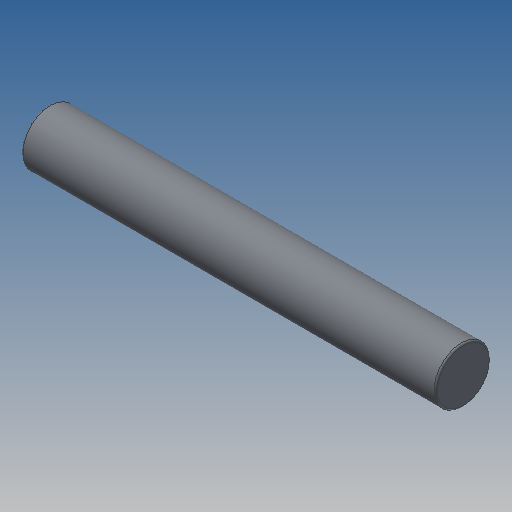
# Autodesk Inventor part: 87994-LtBluishGray
Saved by Autodesk Inventor 2022.2 (Build 262287010, 287A)
## iProperties
Created: 2014-06-03
Part Number: 87994-LtBluishGray
Material: ABS Plastic
Document SubType Name: Modeling
Designer: D. Kohfeld
Appearance: LtBluishGray
Mass: 0.204556 g
Surface Area: 2.56487 cm^2
Volume: 0.192977 cm^3
Density: 1.06 g/cm^3
Author: D. Kohfeld
Autodesk Inventor part; units mm, degrees
ref_plane "YZ Plane" through (0, 0, 0) normal (1, 0, 0) x (0, 1, 0)
ref_plane "XZ Plane" through (0, 0, 0) normal (0, 1, 0) x (-1, 0, 0)
ref_plane "XY Plane" through (0, 0, 0) normal (0, 0, 1) x (1, 0, 0)
sketch "Sketch1" plane through (0, 0, 0) normal (1, 0, 0) x (0, 1, 0)
  circle A0 centre (0, 0) radius 1.6
  dimension "d26" = 3.2
  constraints: 1 centre point, 1 coincident
  measures "d26" diameter of A0
extrude "Extrusion7" add sketch "Sketch1" along normal mid plane 24
fillet "Fillet2" radius 0.1 2 edges at (12, -1.6, 0) (-12, -1.6, 0)
equation "\"d26\" = rd"
equation "\"d27\" = 3 * lu"
equation "\"rd\" = 3.2"
equation "\"lu\" = 8"
body "Solid2"
